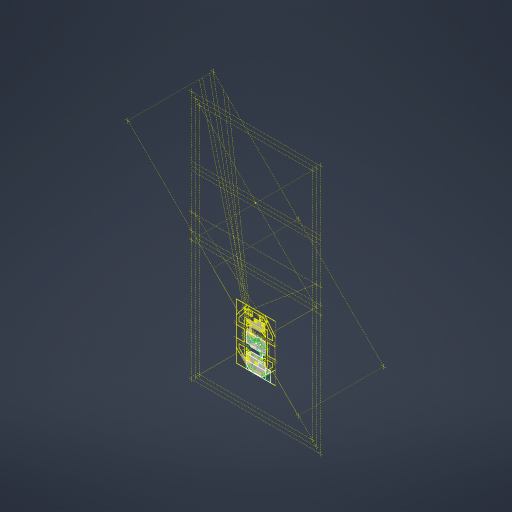
# Autodesk Inventor part: circuit
Saved by Autodesk Inventor 2023.5 (Build 275446000, 446)
## iProperties
Created: 2025-01-19
Part Number: circuit
Material: 一般
Document SubType Name: Modeling
Designer: IshiiLabHonda
Density: 1 g/cm^3
Appearance: 既定
Author: IshiiLabHonda
Autodesk Inventor part; units mm, degrees
ref_plane "YZ Plane" through (0, 0, 0) normal (1, 0, 0) x (0, 1, 0)
ref_plane "XZ Plane" through (0, 0, 0) normal (0, 1, 0) x (-1, 0, 0)
ref_plane "XY Plane" through (0, 0, 0) normal (0, 0, 1) x (1, 0, 0)
derived "chassis.ipt"
sketch "スケッチ1" plane through (0, 0, 0) normal (0, 0, 1) x (1, 0, 0)
  line L0 (-90, 90) -> (90, 90) construction
  line L1 (90, 90) -> (90, -90) construction
  line L2 (90, -90) -> (-90, -90) construction
  line L3 (-90, -90) -> (-90, 90) construction
  line L4 (-90, 90) -> (-90, 270) construction
  line L5 (-90, 270) -> (90, 270) construction
  line L6 (90, 270) -> (90, 90) construction
  line L7 (-90, 90) -> (90, -90) construction
  line L8 (90, 90) -> (-90, -90) construction
  line L9 (0, 0) -> (0, 10) construction
  line L10 (0, 0) -> (10, 0) construction
  line L11 (-90, 270) -> (90, 90) construction
  line L12 (-90, 90) -> (90, 270) construction
  line L13 (-96, 276) -> (96, 276) construction
  line L14 (96, 276) -> (96, -96) construction
  line L15 (96, -96) -> (-96, -96) construction
  line L16 (-96, -96) -> (-96, 276) construction
  line L17 (-84, 264) -> (84, 264) construction
  line L18 (84, 264) -> (84, -84) construction
  line L19 (84, -84) -> (-84, -84) construction
  line L20 (-84, -84) -> (-84, 264) construction
  line L21 (-96, 96) -> (96, 96) construction
  line L22 (-96, 84) -> (96, 84) construction
  line L23 (-63.6396, 63.6396) -> (63.6396, 190.9188) construction
  line L24 (63.6396, 190.9188) -> (190.9188, 63.6396) construction
  line L25 (190.9188, 63.6396) -> (63.6396, -63.6396) construction
  line L26 (63.6396, -63.6396) -> (-63.6396, 63.6396) construction
  line L27 (-190.9188, 190.9188) -> (-63.6396, 318.1981) construction
  line L28 (-63.6396, 318.1981) -> (63.6396, 190.9188) construction
  line L29 (-63.6396, 63.6396) -> (-190.9188, 190.9188) construction
  line L30 (-96, 120) -> (96, 120) construction
  line L31 (-96, 186) -> (96, 186) construction
  line L32 (-96, 174) -> (96, 174) construction
  line L33 (-96, 180) -> (96, 180) construction
  point P0 (-63.6396, 318.1981)
  point P1 (-90, 120)
  point P2 (90, 120)
  point P3 (0, 180)
sketch "スケッチ2" plane through (0, 0, 0) normal (0, 0, 1) x (1, 0, 0)
  line L0 (63.6396, 190.9188) -> (190.9188, 63.6396) construction
  line L1 (-63.6396, 318.1981) -> (63.6396, 190.9188) construction
  line L2 (-84, 264) -> (84, 264) construction
  line L3 (-90, 270) -> (90, 270) construction
  line L4 (90, 270) -> (90, 90) construction
  line L5 (-96, 276) -> (96, 276) construction
  line L6 (-90, 90) -> (90, 270) construction
  line L7 (-90, 270) -> (90, 90) construction
  line L8 (-63.6396, 63.6396) -> (63.6396, 190.9188) construction
  line L9 (-96, 120) -> (96, 120) construction
  line L10 (-90, 90) -> (90, 90) construction
  line L11 (-96, 96) -> (96, 96) construction
  line L12 (-96, 84) -> (96, 84) construction
  line L13 (90, -90) -> (-90, -90) construction
  line L14 (0, 0) -> (0, 10) construction
  line L15 (0, 0) -> (10, 0) construction
  line L16 (190.9188, 63.6396) -> (63.6396, -63.6396) construction
  line L17 (63.6396, -63.6396) -> (-63.6396, 63.6396) construction
  line L18 (84, -84) -> (-84, -84) construction
  line L19 (96, -96) -> (-96, -96) construction
  line L20 (-90, 90) -> (-90, 270) construction
  line L21 (-63.6396, 63.6396) -> (-190.9188, 190.9188) construction
  line L22 (-190.9188, 190.9188) -> (-63.6396, 318.1981) construction
  line L23 (96, 276) -> (96, -96) construction
  line L24 (-96, -96) -> (-96, 276) construction
  line L25 (84, 264) -> (84, -84) construction
  line L26 (-84, -84) -> (-84, 264) construction
  line L27 (90, 90) -> (90, -90) construction
  line L28 (-90, 90) -> (90, -90) construction
  line L29 (90, 90) -> (-90, -90) construction
  line L30 (-90, -90) -> (-90, 90) construction
  circle A0 centre (0, 0) radius 16.5 construction
  circle A1 centre (0, 0) radius 10 construction
  line L31 (20, 11.5) -> (28.75, 11.5) construction
  line L32 (28.75, 11.5) -> (28.75, -11.5) construction
  line L33 (28.75, -11.5) -> (20, -11.5) construction
  line L34 (20, -11.5) -> (20, 11.5) construction
  line L35 (20, 11.5) -> (18, 11.5) construction
  line L36 (18, 11.5) -> (18, -11.5) construction
  line L37 (18, -11.5) -> (20, -11.5) construction
  line L38 (18, 1.5) -> (17, 1.5) construction
  line L39 (17, -1.5) -> (18, -1.5) construction
  line L40 (-17, 24) -> (17, 24) construction
  line L41 (17, 24) -> (17, -24) construction
  line L42 (17, -24) -> (-17, -24) construction
  line L43 (-17, -24) -> (-17, 24) construction
  line L44 (-20, 11.5) -> (-18, 11.5) construction
  line L45 (-17, -1.5) -> (-18, -1.5) construction
  line L46 (-20, -11.5) -> (-20, 11.5) construction
  line L47 (-18, 11.5) -> (-18, -11.5) construction
  line L48 (-28.75, -11.5) -> (-20, -11.5) construction
  line L49 (-20, 11.5) -> (-28.75, 11.5) construction
  line L50 (-28.75, 11.5) -> (-28.75, -11.5) construction
  line L51 (-18, -11.5) -> (-20, -11.5) construction
  line L52 (-18, 1.5) -> (-17, 1.5) construction
  line L53 (-14.5, 24) -> (-14.5, -24) construction
  line L54 (14.5, 24) -> (14.5, -24) construction
  line L55 (-10.5, 24) -> (-10.5, 19) construction
  line L56 (-10.5, 19) -> (-14.5, 19) construction
  line L57 (-14.5, 24) -> (-10.5, 19) construction
  line L58 (-10.5, 24) -> (-14.5, 19) construction
  circle A2 centre (-12.5, 21.5) radius 1 construction
  line L59 (10.5, 24) -> (10.5, 19) construction
  line L60 (10.5, 19) -> (14.5, 19) construction
  line L61 (10.5, 24) -> (14.5, 19) construction
  line L62 (10.5, 19) -> (14.5, 24) construction
  circle A3 centre (12.5, 21.5) radius 1 construction
  line L63 (-14.5, -19) -> (-10.5, -19) construction
  line L64 (-10.5, -19) -> (-10.5, -24) construction
  line L65 (10.5, -24) -> (10.5, -19) construction
  line L66 (10.5, -19) -> (14.5, -19) construction
  line L67 (-14.5, -19) -> (-10.5, -24) construction
  line L68 (-10.5, -19) -> (-14.5, -24) construction
  circle A4 centre (-12.5, -21.5) radius 1 construction
  line L69 (10.5, -19) -> (14.5, -24) construction
  line L70 (14.5, -19) -> (10.5, -24) construction
  circle A5 centre (12.5, -21.5) radius 1 construction
  point P0 (90, 120)
  point P1 (-90, 120)
  point P2 (-63.6396, 318.1981)
  point P3 (-12.5, -21.5)
  point P4 (-12.5, 21.5)
sketch "スケッチ3" plane through (0, 0, 0) normal (0, 0, 1) x (1, 0, 0)
  line L0 (63.6396, 190.9188) -> (190.9188, 63.6396) construction
  line L1 (-63.6396, 318.1981) -> (63.6396, 190.9188) construction
  line L2 (-84, 264) -> (84, 264) construction
  line L3 (-90, 270) -> (90, 270) construction
  line L4 (90, 270) -> (90, 90) construction
  line L5 (-96, 276) -> (96, 276) construction
  line L6 (-90, 90) -> (90, 270) construction
  line L7 (-90, 270) -> (90, 90) construction
  line L8 (-63.6396, 63.6396) -> (63.6396, 190.9188) construction
  line L9 (-96, 120) -> (96, 120) construction
  line L10 (-90, 90) -> (90, 90) construction
  line L11 (-96, 96) -> (96, 96) construction
  line L12 (-96, 84) -> (96, 84) construction
  line L13 (90, -90) -> (-90, -90) construction
  line L14 (0, 0) -> (0, 10) construction
  line L15 (0, 0) -> (10, 0) construction
  line L16 (190.9188, 63.6396) -> (63.6396, -63.6396) construction
  line L17 (63.6396, -63.6396) -> (-63.6396, 63.6396) construction
  line L18 (84, -84) -> (-84, -84) construction
  line L19 (96, -96) -> (-96, -96) construction
  line L20 (-90, 90) -> (-90, 270) construction
  line L21 (-63.6396, 63.6396) -> (-190.9188, 190.9188) construction
  line L22 (-190.9188, 190.9188) -> (-63.6396, 318.1981) construction
  line L23 (96, 276) -> (96, -96) construction
  line L24 (-96, -96) -> (-96, 276) construction
  line L25 (84, 264) -> (84, -84) construction
  line L26 (-84, -84) -> (-84, 264) construction
  line L27 (90, 90) -> (90, -90) construction
  line L28 (-90, 90) -> (90, -90) construction
  line L29 (90, 90) -> (-90, -90) construction
  line L30 (-90, -90) -> (-90, 90) construction
  line L31 (-18, 1.5) -> (-17, 1.5) construction
  line L32 (-17, -1.5) -> (-18, -1.5) construction
  line L33 (-20, 11.5) -> (-18, 11.5) construction
  line L34 (-28.75, 11.5) -> (-28.75, -11.5) construction
  line L35 (63.6396, -63.6396) -> (-63.6396, 63.6396) construction
  line L36 (84, -84) -> (-84, -84) construction
  line L37 (-90, -90) -> (-90, 90) construction
  line L38 (96, -96) -> (-96, -96) construction
  line L39 (-90, 90) -> (90, 90) construction
  line L40 (90, -90) -> (-90, -90) construction
  line L41 (90, 90) -> (-90, -90) construction
  line L42 (-90, 90) -> (90, -90) construction
  line L43 (90, 90) -> (90, -90) construction
  line L44 (-28.75, -11.5) -> (-20, -11.5) construction
  line L45 (-20, 11.5) -> (-28.75, 11.5) construction
  line L46 (-18, 11.5) -> (-18, -11.5) construction
  line L47 (-18, -11.5) -> (-20, -11.5) construction
  line L48 (0, 0) -> (0, 10) construction
  line L49 (0, 0) -> (10, 0) construction
  circle A0 centre (0, 0) radius 16.5 construction
  circle A1 centre (0, 0) radius 10 construction
  line L50 (-14.5, 24) -> (-14.5, -24) construction
  line L51 (-17, 24) -> (17, 24) construction
  line L52 (-17, -24) -> (-17, 24) construction
  line L53 (17, -24) -> (-17, -24) construction
  line L54 (-14.5, -19) -> (-10.5, -19) construction
  circle A2 centre (-12.5, -21.5) radius 1 construction
  line L55 (-10.5, -19) -> (-14.5, -24) construction
  line L56 (-14.5, -19) -> (-10.5, -24) construction
  line L57 (-63.6396, 318.1981) -> (63.6396, 190.9188) construction
  line L58 (-84, 264) -> (84, 264) construction
  line L59 (-90, 270) -> (90, 270) construction
  line L60 (90, 270) -> (90, 90) construction
  line L61 (-96, 276) -> (96, 276) construction
  line L62 (-90, 90) -> (90, 270) construction
  line L63 (-90, 270) -> (90, 90) construction
  line L64 (-63.6396, 63.6396) -> (63.6396, 190.9188) construction
  line L65 (-96, 120) -> (96, 120) construction
  line L66 (-96, 96) -> (96, 96) construction
  line L67 (-96, 84) -> (96, 84) construction
  line L68 (84, 264) -> (84, -84) construction
  line L69 (96, 276) -> (96, -96) construction
  line L70 (-96, -96) -> (-96, 276) construction
  line L71 (-84, -84) -> (-84, 264) construction
  line L72 (-63.6396, 63.6396) -> (-190.9188, 190.9188) construction
  line L73 (-90, 90) -> (-90, 270) construction
  line L74 (-190.9188, 190.9188) -> (-63.6396, 318.1981) construction
  line L75 (-20, -11.5) -> (-20, 11.5) construction
  line L76 (10.5, -19) -> (14.5, -19) construction
  line L77 (10.5, -24) -> (10.5, -19) construction
  circle A3 centre (12.5, -21.5) radius 1 construction
  line L78 (10.5, -19) -> (14.5, -24) construction
  line L79 (14.5, -19) -> (10.5, -24) construction
  line L80 (-10.5, -19) -> (-10.5, -24) construction
  line L81 (63.6396, 190.9188) -> (190.9188, 63.6396) construction
  line L82 (190.9188, 63.6396) -> (63.6396, -63.6396) construction
  line L83 (20, 11.5) -> (28.75, 11.5) construction
  line L84 (28.75, 11.5) -> (28.75, -11.5) construction
  line L85 (17, -1.5) -> (18, -1.5) construction
  line L86 (18, -11.5) -> (20, -11.5) construction
  line L87 (28.75, -11.5) -> (20, -11.5) construction
  line L88 (14.5, 24) -> (14.5, -24) construction
  line L89 (17, 24) -> (17, -24) construction
  line L90 (18, 11.5) -> (18, -11.5) construction
  line L91 (20, -11.5) -> (20, 11.5) construction
  line L92 (20, 11.5) -> (18, 11.5) construction
  line L93 (18, 1.5) -> (17, 1.5) construction
  line L94 (-10.5, 24) -> (-10.5, 19) construction
  line L95 (10.5, 19) -> (14.5, 19) construction
  circle A4 centre (12.5, 21.5) radius 1 construction
  line L96 (10.5, 24) -> (14.5, 19) construction
  line L97 (10.5, 19) -> (14.5, 24) construction
  line L98 (10.5, 24) -> (10.5, 19) construction
  line L99 (-10.5, 19) -> (-14.5, 19) construction
  circle A5 centre (-12.5, 21.5) radius 1 construction
  line L100 (-14.5, 24) -> (-10.5, 19) construction
  line L101 (-10.5, 24) -> (-14.5, 19) construction
  line L102 (29.25, 41.5) -> (29.25, -41.5) construction
  line L103 (29.25, -41.5) -> (-29.25, -41.5) construction
  line L104 (-29.25, -41.5) -> (-29.25, 41.5) construction
  line L105 (-29.25, 8.5) -> (-17, 8.5) construction
  line L106 (-17, 8.5) -> (-17, -8.5) construction
  line L107 (-17, -8.5) -> (-29.25, -8.5) construction
  line L108 (29.25, 8.5) -> (17, 8.5) construction
  line L109 (17, 8.5) -> (17, -8.5) construction
  line L110 (17, -8.5) -> (29.25, -8.5) construction
  line L111 (-2.7087, 12.8503) -> (-1.1893, 4.2332) construction
  line L112 (6.7279, 35.5721) -> (9.9419, 39.4023) construction
  line L113 (5.5106, 35.2882) -> (10.0101, 40.6505) construction
  line L114 (10.4899, 31.11) -> (5.5106, 35.2882) construction
  line L115 (10.0101, 40.6505) -> (10.4899, 31.11) construction
  line L116 (10.5581, 32.3582) -> (9.9419, 39.4023) construction
  line L117 (10.5581, 32.3582) -> (6.7279, 35.5721) construction
  line L118 (10.4899, 31.11) -> (12.788, 29.1817) construction
  line L119 (9.9419, 39.4023) -> (13.7721, 36.1884) construction
  line L120 (6.7279, 35.5721) -> (13.7721, 36.1884) construction
  line L121 (13.7721, 36.1884) -> (10.5581, 32.3582) construction
  line L122 (5.5106, 35.2882) -> (14.9894, 36.4724) construction
  line L123 (10.0101, 40.6505) -> (14.9894, 36.4724) construction
  line L124 (14.9894, 36.4724) -> (10.4899, 31.11) construction
  line L125 (12.788, 29.1817) -> (17.2875, 34.544) construction
  line L126 (17.2875, 34.544) -> (14.9894, 36.4724) construction
  line L127 (-3.5633, 11.938) -> (-2.695, 7.014) construction
  line L128 (-8.4873, 11.0698) -> (-2.695, 7.014) construction
  line L129 (-7.6191, 6.1457) -> (-3.5633, 11.938) construction
  line L130 (-9.1099, 11.7216) -> (-2.7087, 12.8503) construction
  line L131 (-7.6191, 6.1457) -> (-8.4873, 11.0698) construction
  line L132 (-1.1893, 4.2332) -> (-7.5905, 3.1045) construction
  line L133 (-7.5905, 3.1045) -> (-9.1099, 11.7216) construction
  line L134 (-63.6396, 318.1981) -> (-5.5912, 9.0419) construction
  line L135 (10.25, 35.8803) -> (-90, 120) construction
  line L136 (-5.5912, 9.0419) -> (-79.4589, 302.3788) construction
  line L137 (-5.5912, 9.0419) -> (-41.5175, 296.076) construction
  line L138 (-10.25, 35.8803) -> (90, 120) construction
  line L139 (-9.9419, 39.4023) -> (-6.7279, 35.5721) construction
  line L140 (-10.0101, 40.6505) -> (-5.5106, 35.2882) construction
  line L141 (-14.9894, 36.4724) -> (-10.0101, 40.6505) construction
  line L142 (-5.5106, 35.2882) -> (-14.9894, 36.4724) construction
  line L143 (-13.7721, 36.1884) -> (-6.7279, 35.5721) construction
  line L144 (-13.7721, 36.1884) -> (-9.9419, 39.4023) construction
  line L145 (-14.9894, 36.4724) -> (-17.2875, 34.544) construction
  line L146 (-6.7279, 35.5721) -> (-10.5581, 32.3582) construction
  line L147 (-9.9419, 39.4023) -> (-10.5581, 32.3582) construction
  line L148 (-10.0101, 40.6505) -> (-10.4899, 31.11) construction
  line L149 (-5.5106, 35.2882) -> (-10.4899, 31.11) construction
  line L150 (-10.4899, 31.11) -> (-14.9894, 36.4724) construction
  line L151 (-17.2875, 34.544) -> (-12.788, 29.1817) construction
  line L152 (-12.788, 29.1817) -> (-10.4899, 31.11) construction
  line L153 (-10.5581, 32.3582) -> (-13.7721, 36.1884) construction
  circle A6 centre (-7.0361, 32.05) radius 0.625 construction
  circle A7 centre (-7.0361, 32.05) radius 0.8 construction
  circle A8 centre (-7.0361, 32.05) radius 1.5 construction
  circle A9 centre (-16.0715, 34.6506) radius 1.5 construction
  circle A10 centre (-16.0715, 34.6506) radius 0.8 construction
  circle A11 centre (-16.0715, 34.6506) radius 0.625 construction
  line L154 (-2.695, 7.014) -> (-7.6191, 6.1457) construction
  line L155 (-7.9812, 5.3203) -> (-1.58, 6.449) construction
  line L156 (-8.0532, 8.6078) -> (-3.1291, 9.476) construction
  line L157 (-4.6361, 3.6254) -> (-5.157, 6.5799) construction
  line L158 (-8.4873, 11.0698) -> (-3.5633, 11.938) construction
  circle A12 centre (16.0715, 34.6506) radius 1.5 construction
  circle A13 centre (16.0715, 34.6506) radius 0.625 construction
  circle A14 centre (16.0715, 34.6506) radius 0.8
  circle A15 centre (7.0361, 32.05) radius 1.5 construction
  circle A16 centre (7.0361, 32.05) radius 0.8
  circle A17 centre (7.0361, 32.05) radius 0.625 construction
  line L159 (-29.25, -41.5) -> (29.25, -41.5)
  line L160 (-29.25, 41.5) -> (29.25, 41.5)
  line L161 (-10.25, 35.8803) -> (-7.0361, 32.05) construction
  line L162 (-29.25, 20.8653) -> (-13.3068, 41.5)
  line L163 (-29.25, -21.1569) -> (-8.9069, -41.5)
  line L164 (29.25, 20.8653) -> (13.3068, 41.5)
  line L165 (29.25, -21.1569) -> (8.9069, -41.5)
  line L166 (25.25, 19.5) -> (25.25, 14.5)
  line L167 (25.25, 14.5) -> (17, 14.5)
  line L168 (-17, 14.5) -> (-25.25, 14.5)
  line L169 (-25.25, 14.5) -> (-25.25, 19.5)
  line L170 (1.1893, 4.2332) -> (7.5905, 3.1045) construction
  line L171 (7.5905, 3.1045) -> (9.1099, 11.7216) construction
  line L172 (2.7087, 12.8503) -> (1.1893, 4.2332) construction
  line L173 (2.695, 7.014) -> (7.6191, 6.1457) construction
  line L174 (7.9812, 5.3203) -> (1.58, 6.449) construction
  line L175 (8.4873, 11.0698) -> (2.695, 7.014) construction
  line L176 (7.6191, 6.1457) -> (3.5633, 11.938) construction
  line L177 (3.5633, 11.938) -> (2.695, 7.014) construction
  line L178 (8.4873, 11.0698) -> (3.5633, 11.938) construction
  line L179 (7.6191, 6.1457) -> (8.4873, 11.0698) construction
  line L180 (9.1099, 11.7216) -> (2.7087, 12.8503) construction
  line L181 (13.5, 30) -> (13.5, 24)
  line L182 (13.5, 24) -> (17, 24)
  line L183 (17, 24) -> (17, 14.5)
  line L184 (-13.5, 24) -> (-17, 24)
  line L185 (-17, 24) -> (-17, 14.5)
  line L186 (-17, -14.5) -> (-25.25, -14.5)
  line L187 (-25.25, -14.5) -> (-25.25, -19.5)
  line L188 (-25.25, -19.5) -> (-7.25, -37.5)
  line L189 (-7.25, -37.5) -> (7.25, -37.5)
  line L190 (7.25, -37.5) -> (25.25, -19.5)
  line L191 (25.25, -19.5) -> (25.25, -14.5)
  line L192 (25.25, -14.5) -> (17, -14.5)
  line L193 (17, -14.5) -> (17, -24)
  line L194 (17, -24) -> (13.5, -24)
  line L195 (-13.5, -30) -> (-13.5, -24)
  line L196 (-13.5, -24) -> (-17, -24)
  line L197 (-17, -24) -> (-17, -14.5)
  line L198 (-9.1099, 11.7216) -> (-7.5905, 3.1045) construction
  line L199 (-9.4721, 10.8961) -> (-8.6039, 5.9721) construction
  line L200 (-14.3961, 10.0279) -> (-8.6039, 5.9721) construction
  line L201 (-13.5279, 5.1039) -> (-9.4721, 10.8961) construction
  line L202 (-13.5279, 5.1039) -> (-14.3961, 10.0279) construction
  line L203 (-7.5905, 3.1045) -> (-13.9918, 1.9758) construction
  line L204 (-14.3961, 10.0279) -> (-9.4721, 10.8961) construction
  line L205 (-13.962, 7.5659) -> (-9.038, 8.4341) construction
  line L206 (-8.6039, 5.9721) -> (-13.5279, 5.1039) construction
  line L207 (-10.5449, 2.5836) -> (-11.0659, 5.538) construction
  line L208 (-15.5112, 10.5929) -> (-9.1099, 11.7216) construction
  line L209 (9.4721, 10.8961) -> (8.6039, 5.9721) construction
  line L210 (9.1099, 11.7216) -> (7.5905, 3.1045) construction
  line L211 (14.3961, 10.0279) -> (9.4721, 10.8961) construction
  line L212 (13.962, 7.5659) -> (9.038, 8.4341) construction
  line L213 (10.5449, 2.5836) -> (11.0659, 5.538) construction
  line L214 (15.5112, 10.5929) -> (9.1099, 11.7216) construction
  line L215 (13.5279, 5.1039) -> (9.4721, 10.8961) construction
  line L216 (8.6039, 5.9721) -> (13.5279, 5.1039) construction
  line L217 (14.3961, 10.0279) -> (8.6039, 5.9721) construction
  line L218 (13.5279, 5.1039) -> (14.3961, 10.0279) construction
  line L219 (13.9918, 1.9758) -> (15.5112, 10.5929) construction
  line L220 (7.5905, 3.1045) -> (13.9918, 1.9758) construction
  line L221 (-25.25, 19.5) -> (-11.3425, 37.5)
  line L222 (-11.3425, 37.5) -> (11.3425, 37.5)
  line L223 (11.3425, 37.5) -> (25.25, 19.5)
  circle A18 centre (0, 0) radius 4.25 construction
  line L224 (-11.5, 8) -> (-68.7791, 313.0586) construction
  line L225 (-11.5, 8) -> (-84.3887, 297.449) construction
  line L226 (-11.5, 8) -> (-48.4208, 302.9793) construction
  line L227 (-15.5112, 10.5929) -> (-13.9918, 1.9758) construction
  line L228 (-14.3825, 4.1916) -> (-7.9812, 5.3203) construction
  circle A19 centre (-10.5, -27) radius 1
  circle A20 centre (10.5, 27) radius 1
  circle A21 centre (10.5, 27) radius 2
  circle A22 centre (-10.5, -27) radius 2
  circle A23 centre (0, -27) radius 1
  circle A24 centre (0, -27) radius 2
  circle A25 centre (0, 27) radius 1
  circle A26 centre (0, 27) radius 2
  line L229 (0, 27) -> (10.5, 27) construction
  line L230 (-10.5, -27) -> (0, -27) construction
  line L231 (13.5, 30) -> (-3, 30)
  line L232 (-3, 30) -> (-3, 24)
  line L233 (-13.5, 24) -> (-3, 24)
  line L234 (-13.5, -30) -> (3, -30)
  line L235 (3, -30) -> (3, -24)
  line L236 (3, -24) -> (13.5, -24)
  line L237 (-16.1606, 31.2641) -> (-6.1594, 29.9135)
  line L238 (-6.1594, 29.9135) -> (-5.0634, 31.332)
  line L239 (-5.0634, 31.332) -> (-4.8147, 37.5)
  line L240 (6.1594, 29.9135) -> (5.0634, 31.332)
  line L241 (16.1606, 31.2641) -> (6.1594, 29.9135)
  line L242 (5.0634, 31.332) -> (4.8147, 37.5)
  line L243 (-10.5, -27) -> (-14.125, -30.625) construction
  line L244 (-15.5392, -29.2108) -> (-13.5, -24)
  line L245 (-12.7108, -32.0392) -> (-7.5, -30)
  line L246 (10.5, 27) -> (13.5, 30) construction
  line L247 (16.1606, 31.2641) -> (10.0926, 30)
  line L248 (-10.5, -19) -> (-10.5, -20.4081)
  line L249 (-10.5, -20.4081) -> (-7.5, -21.5)
  line L250 (-7.5, -21.5) -> (7.5, -21.5)
  line L251 (7.5, -21.5) -> (10.5, -20.4081)
  line L252 (10.5, -20.4081) -> (10.5, -19)
  line L253 (10.5, -19) -> (-10.5, -19)
  line L254 (7.5, 21.5) -> (10.5, 20.4081)
  line L255 (10.5, 20.4081) -> (10.5, 19)
  line L256 (-7.5, 21.5) -> (7.5, 21.5)
  line L257 (10.5, 19) -> (-10.5, 19)
  line L258 (-10.5, 19) -> (-10.5, 20.4081)
  line L259 (-10.5, 20.4081) -> (-7.5, 21.5)
  line L260 (-5.3602, -19) -> (-14.5, -13.3971)
  line L261 (-14.5, -13.3971) -> (-14.5, -15.3971)
  line L262 (0, 0) -> (-9.9301, -16.1985) construction
  line L263 (14.5, -13.3971) -> (14.5, -15.3971)
  line L264 (5.3602, -19) -> (14.5, -13.3971)
  line L265 (-5.3602, 19) -> (-14.5, 13.3971)
  line L266 (-14.5, 13.3971) -> (-14.5, 15.3971)
  line L267 (5.3602, 19) -> (14.5, 13.3971)
  line L268 (14.5, 13.3971) -> (14.5, 15.3971)
  line L269 (-14.5, -15.3971) -> (-10.5, -20.4081)
  line L270 (10.5, -20.4081) -> (14.5, -15.3971)
  line L271 (-14.5, 15.3971) -> (-10.5, 20.4081)
  line L272 (14.5, 15.3971) -> (10.5, 20.4081)
  line L273 (-5.3602, -19) -> (-9.4462, -17.5128)
  line L274 (-9.4462, -17.5128) -> (-14.5, -13.3971)
  line L275 (-10.5, -20.4081) -> (-9.4462, -17.5128) construction
  line L276 (9.4462, -17.5128) -> (14.5, -13.3971)
  line L277 (5.3602, -19) -> (9.4462, -17.5128)
  line L278 (-5.3602, 19) -> (-9.4462, 17.5128)
  line L279 (-9.4462, 17.5128) -> (-14.5, 13.3971)
  line L280 (9.4462, 17.5128) -> (14.5, 13.3971)
  line L281 (5.3602, 19) -> (9.4462, 17.5128)
  point P0 (90, 120)
  point P1 (90, 120)
  point P2 (11.5, 8)
  point P3 (11.5, 8)
  point P4 (-5.5912, 9.0419)
  point P5 (-5.5912, 9.0419)
  point P6 (13.6038, 24)
  point P7 (6.0926, 30)
  dimension "d60" = 20
  measures "d60" diameter of A1
sketch "スケッチ4" plane through (0, 0, 0) normal (0, 0, 1) x (1, 0, 0)
  line L0 (0, 0) -> (0, 10) construction
  line L1 (0, 0) -> (10, 0) construction
  line L2 (0, 0) -> (0, 10) construction
  circle A0 centre (0, 0) radius 10 construction
  line L3 (-17, -24) -> (-17, 24) construction
  line L4 (-14.5, 24) -> (-14.5, -24) construction
  line L5 (17, -24) -> (-17, -24) construction
  circle A1 centre (0, 0) radius 16.5 construction
  line L6 (0, 0) -> (10, 0) construction
  line L7 (17, -1.5) -> (18, -1.5) construction
  line L8 (14.5, 24) -> (14.5, -24) construction
  line L9 (17, 24) -> (17, -24) construction
  line L10 (18, 1.5) -> (17, 1.5) construction
  line L11 (18, -11.5) -> (20, -11.5) construction
  line L12 (18, 11.5) -> (18, -11.5) construction
  line L13 (20, -11.5) -> (20, 11.5) construction
  line L14 (20, 11.5) -> (18, 11.5) construction
  line L15 (-18, 11.5) -> (-18, -11.5) construction
  line L16 (-20, -11.5) -> (-20, 11.5) construction
  line L17 (-18, 1.5) -> (-17, 1.5) construction
  line L18 (-17, -1.5) -> (-18, -1.5) construction
  line L19 (-18, -11.5) -> (-20, -11.5) construction
  line L20 (28.75, 11.5) -> (28.75, -11.5) construction
  line L21 (28.75, -11.5) -> (20, -11.5) construction
  line L22 (20, 11.5) -> (28.75, 11.5) construction
  line L23 (-17, 24) -> (17, 24) construction
  line L24 (-20, 11.5) -> (-18, 11.5) construction
  line L25 (-20, 11.5) -> (-28.75, 11.5) construction
  line L26 (-28.75, 11.5) -> (-28.75, -11.5) construction
  line L27 (-28.75, -11.5) -> (-20, -11.5) construction
  line L28 (10.5, -19) -> (14.5, -19) construction
  circle A2 centre (12.5, -21.5) radius 1 construction
  line L29 (10.5, -19) -> (14.5, -24) construction
  line L30 (14.5, -19) -> (10.5, -24) construction
  line L31 (10.5, -24) -> (10.5, -19) construction
  line L32 (-14.5, -19) -> (-10.5, -19) construction
  line L33 (-10.5, -19) -> (-10.5, -24) construction
  line L34 (-14.5, -19) -> (-10.5, -24) construction
  line L35 (-10.5, -19) -> (-14.5, -24) construction
  circle A3 centre (-12.5, -21.5) radius 1 construction
  line L36 (-10.5, 19) -> (-14.5, 19) construction
  circle A4 centre (-12.5, 21.5) radius 1 construction
  line L37 (-14.5, 24) -> (-10.5, 19) construction
  line L38 (-10.5, 24) -> (-14.5, 19) construction
  line L39 (10.5, 19) -> (14.5, 19) construction
  line L40 (10.5, 24) -> (10.5, 19) construction
  circle A5 centre (12.5, 21.5) radius 1 construction
  line L41 (10.5, 24) -> (14.5, 19) construction
  line L42 (10.5, 19) -> (14.5, 24) construction
  line L43 (-10.5, 24) -> (-10.5, 19) construction
  line L44 (0, 0) -> (0, 10) construction
  line L45 (0, 0) -> (10, 0) construction
  line L46 (10.5, -24) -> (10.5, -19) construction
  line L47 (17, -1.5) -> (18, -1.5) construction
  line L48 (18, 1.5) -> (17, 1.5) construction
  line L49 (20, -11.5) -> (20, 11.5) construction
  line L50 (18, 11.5) -> (18, -11.5) construction
  line L51 (28.75, 11.5) -> (28.75, -11.5) construction
  line L52 (-10.5, -19) -> (-10.5, -24) construction
  line L53 (10.5, 19) -> (14.5, 19) construction
  circle A6 centre (12.5, 21.5) radius 1 projected
  line L54 (-17, -1.5) -> (-18, -1.5) construction
  line L55 (14.5, 24) -> (14.5, -24) construction
  line L56 (10.5, 24) -> (14.5, 19) construction
  line L57 (10.5, 19) -> (14.5, 24) construction
  line L58 (17, 24) -> (17, -24) construction
  line L59 (10.5, 24) -> (10.5, 19) construction
  line L60 (-18, 1.5) -> (-17, 1.5) construction
  line L61 (-17, 8.5) -> (-17, -8.5) projected
  line L62 (-20, 11.5) -> (-18, 11.5) construction
  line L63 (-20, -11.5) -> (-20, 11.5) construction
  line L64 (-29.25, -41.5) -> (-29.25, 41.5) projected
  line L65 (-28.75, 11.5) -> (-28.75, -11.5) construction
  line L66 (18, -11.5) -> (20, -11.5) construction
  line L67 (10.5, -19) -> (14.5, -19) construction
  line L68 (28.75, -11.5) -> (20, -11.5) construction
  line L69 (10.5, -19) -> (14.5, -24) construction
  line L70 (20, 11.5) -> (18, 11.5) construction
  line L71 (29.25, 8.5) -> (17, 8.5) projected
  line L72 (20, 11.5) -> (28.75, 11.5) construction
  line L73 (17, 8.5) -> (17, -8.5) projected
  line L74 (-20, 11.5) -> (-28.75, 11.5) construction
  line L75 (10.0101, 40.6505) -> (14.9894, 36.4724) construction
  line L76 (10.4899, 31.11) -> (12.788, 29.1817) construction
  line L77 (12.788, 29.1817) -> (17.2875, 34.544) construction
  line L78 (10.5581, 32.3582) -> (9.9419, 39.4023) construction
  line L79 (6.7279, 35.5721) -> (9.9419, 39.4023) construction
  line L80 (5.5106, 35.2882) -> (10.0101, 40.6505) construction
  line L81 (10.5581, 32.3582) -> (6.7279, 35.5721) construction
  line L82 (10.4899, 31.11) -> (5.5106, 35.2882) construction
  line L83 (10.0101, 40.6505) -> (10.4899, 31.11) construction
  line L84 (6.7279, 35.5721) -> (13.7721, 36.1884) construction
  line L85 (5.5106, 35.2882) -> (14.9894, 36.4724) construction
  line L86 (9.9419, 39.4023) -> (13.7721, 36.1884) construction
  line L87 (13.7721, 36.1884) -> (10.5581, 32.3582) construction
  line L88 (14.9894, 36.4724) -> (10.4899, 31.11) construction
  line L89 (17.2875, 34.544) -> (14.9894, 36.4724) construction
  circle A7 centre (-12.5, 21.5) radius 1 projected
  line L90 (-10.5, 19) -> (-14.5, 19) construction
  line L91 (-10.5, 24) -> (-10.5, 19) construction
  line L92 (-14.5, 24) -> (-10.5, 19) construction
  line L93 (-10.5, 24) -> (-14.5, 19) construction
  line L94 (-7.6191, 6.1457) -> (-8.4873, 11.0698) construction
  line L95 (-3.5633, 11.938) -> (-2.695, 7.014) construction
  line L96 (-7.6191, 6.1457) -> (-3.5633, 11.938) construction
  line L97 (-8.4873, 11.0698) -> (-2.695, 7.014) construction
  line L98 (-1.1893, 4.2332) -> (-7.5905, 3.1045) construction
  line L99 (-2.7087, 12.8503) -> (-1.1893, 4.2332) construction
  line L100 (-9.1099, 11.7216) -> (-2.7087, 12.8503) construction
  line L101 (-7.5905, 3.1045) -> (-9.1099, 11.7216) construction
  line L102 (-28.75, -11.5) -> (-20, -11.5) construction
  line L103 (-29.25, 8.5) -> (-17, 8.5) projected
  line L104 (-12.788, 29.1817) -> (-10.4899, 31.11) construction
  circle A8 centre (-16.0715, 34.6506) radius 0.625 projected
  circle A9 centre (-16.0715, 34.6506) radius 0.8 construction
  circle A10 centre (-16.0715, 34.6506) radius 1.5 construction
  line L105 (-17.2875, 34.544) -> (-12.788, 29.1817) construction
  line L106 (-5.5106, 35.2882) -> (-10.4899, 31.11) construction
  line L107 (-6.7279, 35.5721) -> (-10.5581, 32.3582) construction
  line L108 (-5.5106, 35.2882) -> (-14.9894, 36.4724) construction
  line L109 (-13.7721, 36.1884) -> (-6.7279, 35.5721) construction
  line L110 (-10.5581, 32.3582) -> (-13.7721, 36.1884) construction
  line L111 (-14.9894, 36.4724) -> (-17.2875, 34.544) construction
  line L112 (-10.4899, 31.11) -> (-14.9894, 36.4724) construction
  line L113 (-13.7721, 36.1884) -> (-9.9419, 39.4023) construction
  line L114 (-9.9419, 39.4023) -> (-10.5581, 32.3582) construction
  line L115 (-14.9894, 36.4724) -> (-10.0101, 40.6505) construction
  line L116 (-10.0101, 40.6505) -> (-10.4899, 31.11) construction
  line L117 (0, 0) -> (0, 10) construction
  line L118 (0, 0) -> (10, 0) construction
  circle A11 centre (0, 0) radius 10 construction
  line L119 (-14.5, -19) -> (-10.5, -19) construction
  circle A12 centre (0, 0) radius 16.5 construction
  circle A13 centre (12.5, -21.5) radius 1 projected
  line L120 (14.5, -19) -> (10.5, -24) construction
  circle A14 centre (-12.5, -21.5) radius 1 projected
  line L121 (-14.5, -19) -> (-10.5, -24) construction
  line L122 (17, -24) -> (-17, -24) construction
  line L123 (29.25, -41.5) -> (-29.25, -41.5) projected
  line L124 (-17, -8.5) -> (-29.25, -8.5) projected
  line L125 (-18, -11.5) -> (-20, -11.5) construction
  line L126 (-18, 11.5) -> (-18, -11.5) construction
  circle A15 centre (-7.0361, 32.05) radius 0.625 projected
  circle A16 centre (-7.0361, 32.05) radius 1.5 construction
  line L127 (-9.9419, 39.4023) -> (-6.7279, 35.5721) construction
  line L128 (-10.0101, 40.6505) -> (-5.5106, 35.2882) construction
  circle A17 centre (-7.0361, 32.05) radius 0.8 construction
  line L129 (-10.5, -19) -> (-14.5, -24) construction
  line L130 (-14.5, 24) -> (-14.5, -24) construction
  line L131 (-17, -24) -> (-17, 24) construction
  line L132 (-17, 24) -> (17, 24) construction
  line L133 (17, -8.5) -> (29.25, -8.5) projected
  line L134 (-14, 7.5) -> (-14, -7.5)
  line L135 (-14, -7.5) -> (14, -7.5)
  line L136 (14, 7.5) -> (14, -7.5)
  circle A18 centre (-7.25, 0) radius 0.8
  circle A19 centre (0, 0) radius 4.25 construction
  circle A20 centre (0, 0) radius 4.3 construction
  circle A21 centre (0, 0) radius 5.75 construction
  circle A22 centre (-7.25, 0) radius 1.5 construction
  circle A23 centre (7.25, 0) radius 1.5 construction
  circle A24 centre (7.25, 0) radius 0.8
  circle A25 centre (0, 0) radius 1.5
  line L137 (-14, 7.5) -> (14, 7.5)
  line L138 (-14, 7.5) -> (-9.5, 7.5)
  line L139 (-6, 7.5) -> (14, 7.5)
  line L140 (6, -7.5) -> (6, -15.5)
  line L141 (6, -15.5) -> (10, -15.5)
  line L142 (10, -15.5) -> (10, -7.5)
  line L143 (-8, -15.5) -> (10, -15.5)
  line L144 (10, -15.5) -> (10, -21.5)
  line L145 (10, -21.5) -> (-8, -21.5)
  line L146 (-8, -21.5) -> (-8, -15.5)
  line L147 (-8, -18.5) -> (-14, -18.5)
  line L148 (-14, -18.5) -> (-14, -21.5)
  line L149 (-14, -21.5) -> (-8, -21.5)
  line L150 (-8, -21.5) -> (-8, -18.5)
  line L151 (-8, -7.5) -> (6, -7.5)
  line L152 (6, -7.5) -> (6, -9.5)
  line L153 (6, -9.5) -> (-8, -9.5)
  line L154 (-8, -9.5) -> (-8, -7.5)
  line L155 (10, -19.5) -> (14, -19.5)
  line L156 (14, -19.5) -> (14, -21.5)
  line L157 (14, -21.5) -> (10, -21.5)
  line L158 (10, -21.5) -> (10, -19.5)
  line L159 (10, -7.5) -> (14, -7.5)
  line L160 (14, -7.5) -> (14, -10.5)
  line L161 (14, -10.5) -> (10, -10.5)
  line L162 (10, -10.5) -> (10, -7.5)
  line L163 (-14, -21.5) -> (14, -21.5)
  line L164 (14, -21.5) -> (14, -30)
  line L165 (14, -30) -> (-14, -30)
  line L166 (-14, -30) -> (-14, -21.5)
  line L167 (-13.5, -30) -> (3, -30) projected
  line L168 (3, -30) -> (3, -24)
  line L169 (3, -24) -> (14, -24)
  line L170 (3, -30) -> (14, -30)
  line L171 (14, -30) -> (14, -24)
  line L172 (-14, -30) -> (-14, -41.5)
  line L173 (-14, -41.5) -> (14, -41.5)
  line L174 (14, -41.5) -> (14, -30)
  line L175 (-29.25, -21.1569) -> (-8.9069, -41.5) projected
  line L176 (29.25, -21.1569) -> (8.9069, -41.5) projected
  line L177 (14, -26) -> (22, -26)
  line L178 (22, -26) -> (22, -41.5)
  line L179 (22, -41.5) -> (14, -41.5)
  line L180 (-14, -35.6997) -> (-8.1997, -41.5)
  line L181 (-9.1997, -40.5) -> (9.9069, -40.5)
  line L182 (8.1997, -41.5) -> (22, -27.6997)
  point P0 (-12.5, -21.5)
  point P1 (-12.5, 21.5)
  point P2 (10.25, 35.8803)
  point P3 (-5.5912, 9.0419)
  point P4 (-10.25, 35.8803)
  point P5 (6, -15.5)
  point P6 (14, -8)
  point P7 (14, -36.4069)
  point P8 (8.9069, -41.5)
  point P9 (-8.9069, -41.5)
  point P10 (-14, -36.4069)
  point P11 (22, -28.4069)
  point P12 (8.1997, -41.5)
  point P13 (9.1997, -40.5)
  dimension "d2" = 0.5
  dimension "d3" = 0.5
  dimension "d4" = 1.6
  dimension "d5" = 8.5
  dimension "d6" = 0.05
  dimension "d8" = 3
  dimension "d9" = 3
  dimension "d10" = 1.6
  dimension "d11" = 3
  dimension "d18" = 7.5
  dimension "d19" = 7.5
  dimension "d20" = 4
  dimension "d21" = 4
  dimension "d22" = 8
  dimension "d26" = 11
  dimension "d27" = 18
  dimension "d28" = 2
  dimension "d29" = 2
  dimension "d30" = 3
  dimension "d61" = 1.5
  dimension "d75" = 11.5
  dimension "d82" = 8
  dimension "d83" = 15.5
  dimension "d84" = 0.5
  dimension "d85" = 1
  dimension "d86" = 0.5
  constraints: 92 end point, 25 point on line, 20 parallel, 13 perpendicular, 8 centre point, 6 coincident, 6 collinear, 5 horizontal, 2 tangent, 1 midpoint, 1 vertical, 19 other
  measures "d2" distance between parallel lines of L4 L134
  measures "d3" distance between parallel lines of L136 L8
  measures "d4" diameter of A18
  measures "d5" diameter of A19
  measures "d6" radial gap between concentric circles of A19 A20
  measures "d8" diameter of A22
  measures "d9" diameter of A23
  measures "d10" diameter of A24
  measures "d11" diameter of A25
  measures "d18" distance of the line from the sketch origin of L139
  measures "d19" distance of the line from the sketch origin of L135
  measures "d20" distance between parallel lines of L140 L142
  measures "d21" distance between parallel lines of L136 L142
  measures "d22" distance between parallel lines of L141 L135
  measures "d26" distance between parallel lines of L147 L135
  measures "d27" distance between parallel lines of L144 L146
  measures "d28" distance between parallel lines of L157 L155
  measures "d29" distance between parallel lines of L153 L135
  measures "d30" distance between parallel lines of L161 L159
  measures "d61" radial gap between concentric circles of A21 A19
  measures "d75" distance between parallel lines of L173 L167
  measures "d82" distance between parallel lines of L178 L174
  measures "d83" distance between parallel lines of L179 L177
  measures "d84" distance between parallel lines of L175 L180
  measures "d85" distance between parallel lines of L173 L181
  measures "d86" distance between parallel lines of L176 L182
extrude "押し出し3" add sketch "スケッチ4" against normal blind 0.8 contours L166 L149 A14 L145 L157 A13 L164 L169 L168 L165 | L148 L147 L146 L149 A14 | L168 L169 L164 L165 | L149 A14 | A14 L149 | L146 L143 L141 L144 L145 | L157 A13 L144 L155 L156 | L140 L135 L142 L141 | L157 A13 | A13 L157 | L153 L154 L135 L140 | L142 L135 L160 L161
extrude "押し出し4" add sketch "スケッチ4" against normal blind 0.8 contours L135 L134 L137 L136
pattern_circular "円形状パターン1" count 2 over 360 about axis through (0, 0, -10) along (0, 0, 1) of "押し出し3"
extrude "押し出し5" cut sketch "スケッチ3" against normal blind 0.8 contours A19 | A20
extrude "押し出し6" cut sketch "スケッチ3" against normal blind 0.8 contours A23 | A25
extrude "押し出し7" cut sketch "スケッチ4" against normal blind 0.8 contours L168 L169 L164 L165
pattern_circular "円形状パターン2" count 2 over 360 about axis through (0, 0, -10) along (0, 0, 1) of "押し出し7"
chamfer "面取り5" distance 0.5 angle 45 12 edges at (-10, 10.5, -0.4) (-10, 19.5, -0.4) (-6, 15.5, -0.4) (-6, 9.5, -0.4) (6, -9.5, -0.4) (6, -15.5, -0.4) (10, -10.5, -0.4) (10, -19.5, -0.4) (8, 18.5, -0.4) (8, 7.5, -0.4) (-8, -7.5, -0.4) (-8, -18.5, -0.4)
extrude "押し出し8" add sketch "スケッチ4" against normal blind 0.8 contours L168 L169 L164 L165
chamfer "面取り7" distance 0.5 angle 45 12 edges at (8, 9.5, -0.4) (14, 7.5, -0.4) (8, 15.5, -0.4) (14, 18.5, -0.4) (14, -10.5, -0.4) (14, -19.5, -0.4) (-14, -18.5, -0.4) (-8, -15.5, -0.4) (-8, -9.5, -0.4) (-14, -7.5, -0.4) (-14, 10.5, -0.4) (-14, 19.5, -0.4)
extrude "押し出し9" add sketch "スケッチ4" against normal blind 0.8 contours L172 L175 L123 | L172 L180 L123 L175 | L172 L165 L174 L182 L181 L180 | L180 L181 L182 L123 | L182 L181 L176 L123 | L182 L174 L176 L181 | L176 L174 L123
extrude "押し出し11" add sketch "スケッチ4" against normal blind 0.8 contours L182 L178 L176 L174 | L174 L164 L177 L178 L182 | L174 L176 L178 L123
extrude "押し出し13" cut sketch "スケッチ4" against normal blind 0.8 contours L172 L175 L123 | L172 L180 L123 L175 | L180 L181 L182 L123
extrude "押し出し14" cut sketch "スケッチ4" against normal blind 0.8 contours L182 L181 L176 L123 | L182 L174 L176 L181 | L176 L174 L123 | L182 L178 L176 L174 | L174 L176 L178 L123
mirror "ミラー2" about plane through (0, 0, 0) normal (1, 0, 0) of "押し出し11", "押し出し14"
chamfer "面取り8" distance 0.5 angle 45 2 edges at (-9.1997, -40.5, -0.4) (9.1997, -40.5, -0.4)
chamfer "面取り9" distance 0.5 angle 45 2 edges at (-22, -26, -0.4) (22, -26, -0.4)
chamfer "面取り10" distance 2 angle 45 2 edges at (-3, 30, -0.4) (14, 30, -0.4)
chamfer "面取り11" distance 0.5 angle 45 2 edges at (-14, 24, -0.4) (-3, 24, -0.4)
